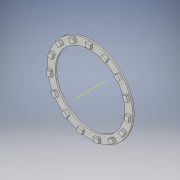
# Autodesk Inventor part: LightRing
Saved by Autodesk Inventor 2019.2 (Build 232265000, 265)
## iProperties
Created: 2019-01-11
Part Number: LightRing
Material: Generic
Document SubType Name: Modeling
Designer: SnoBotics
Density: 1 g/cm^3
Appearance: Default
Author: SnoBotics
Autodesk Inventor part; units mm, degrees
ref_plane "YZ Plane" through (0, 0, 0) normal (1, 0, 0) x (0, 1, 0)
ref_plane "XZ Plane" through (0, 0, 0) normal (0, 1, 0) x (-1, 0, 0)
ref_plane "XY Plane" through (0, 0, 0) normal (0, 0, 1) x (1, 0, 0)
sketch "Sketch1" plane through (0, 0, 0) normal (0, 0, 1) x (1, 0, 0)
  circle A0 centre (0, 0) radius 30
  circle A1 centre (0, 0) radius 24.5
  dimension "d0" = 49
  dimension "d1" = 60
  constraints: 2 centre point, 2 coincident
  measures "d0" diameter of A1
  measures "d1" diameter of A0
extrude "Extrusion1" add sketch "Sketch1" against normal blind 1.1
sketch "Sketch2" plane through (0, 0, 0) normal (0, 0, 1) x (1, 0, 0)
  line L0 (0, 0) -> (0, 30) construction
  circle A0 centre (0, 0) radius 30 construction
  line L1 (-1.7914, 26.2382) -> (1.7914, 26.2382)
  line L2 (1.7914, 26.2382) -> (1.7914, 29.0379)
  line L3 (1.7914, 29.0379) -> (-1.7914, 29.0379)
  line L4 (-1.7914, 29.0379) -> (-1.7914, 26.2382)
  line L5 (-1.7914, 26.2382) -> (1.7914, 29.0379) construction
  line L6 (1.7914, 26.2382) -> (-1.7914, 29.0379) construction
  point P0 (0, 27.6381)
  constraints: 14 end point, 2 midpoint, 2 parallel, 1 horizontal, 1 perpendicular, 1 point on line, 1 vertical, 1 vertical alignment, 1 other
extrude "Extrusion2" add sketch "Sketch2" along normal blind 1.7
pattern_circular "Circular Pattern1" count 15 over 360 about axis through (0, 0, -10) along (0, 0, 1) of "Extrusion2"
body "Solid1"
